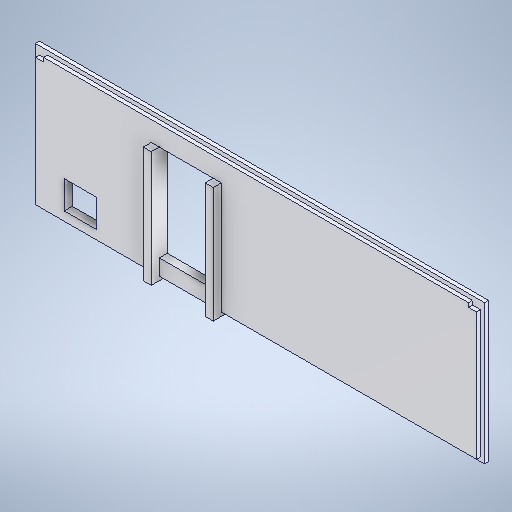
# Autodesk Inventor part: back
Saved by Autodesk Inventor 2025 (Build 290162000, 162)
## iProperties
Created: 2025-05-20
Part Number: back
Material: Generic
Document SubType Name: Modeling
Designer: ethan
Density: 1 g/cm^3
Appearance: PTFE
Author: ethan
Autodesk Inventor part; units mm, degrees
ref_plane "YZ Plane" through (0, 0, 0) normal (1, 0, 0) x (0, 1, 0)
ref_plane "XZ Plane" through (0, 0, 0) normal (0, 1, 0) x (-1, 0, 0)
ref_plane "XY Plane" through (0, 0, 0) normal (0, 0, 1) x (1, 0, 0)
sketch "Sketch1" plane through (0, 0, 0) normal (0, 0, 1) x (1, 0, 0)
  line L0 (0, 0) -> (224.6, 0)
  line L1 (224.6, 0) -> (224.6, 69.85)
  line L2 (224.6, 69.85) -> (0, 69.85)
  line L3 (0, 69.85) -> (0, 0)
  dimension "d0" = 224.6
  dimension "d1" = 69.85
  constraints: 8 end point, 2 parallel, 1 horizontal, 1 perpendicular
  measures "d0" distance of L2.end L1.end
  measures "d1" distance of L1.end L0.end
extrude "Extrusion1" add sketch "Sketch1" along normal blind 2
sketch "Sketch2" plane through (0, 0, 2) normal (0, 0, 1) x (1, 0, 0)
  line L0 (224.6, 0) -> (224.6, 69.85) projected
  line L1 (224.6, 69.85) -> (0, 69.85) projected
  line L2 (0, 69.85) -> (0, 0) projected
  line L3 (0, 0) -> (224.6, 0) projected
  line L4 (2, 67.85) -> (222.6, 67.85)
  line L5 (222.6, 67.85) -> (222.6, 2)
  line L6 (222.6, 2) -> (2, 2)
  line L7 (2, 2) -> (2, 67.85)
  dimension "d4" = 2
  constraints: 8 end point, 3 other
  measures "d4" distance between parallel lines of L1 L4
extrude "Extrusion2" add sketch "Sketch2" along normal blind 2 contours L4 L5 L6 L7
sketch "Sketch3" plane through (0, 0, 4) normal (0, 0, 1) x (1, 0, 0)
  line L0 (2, 2) -> (222.6, 2) construction
  line L1 (222.6, 2) -> (222.6, 67.85) construction
  line L2 (222.6, 67.85) -> (2, 67.85) construction
  line L3 (2, 67.85) -> (2, 2) construction
  line L4 (2, 67.85) -> (6, 67.85)
  line L5 (6, 67.85) -> (6, 65.85)
  line L6 (6, 65.85) -> (2, 65.85)
  line L7 (2, 65.85) -> (2, 67.85)
  line L8 (222.6, 67.85) -> (218.6, 67.85)
  line L9 (218.6, 67.85) -> (218.6, 65.85)
  line L10 (218.6, 65.85) -> (222.6, 65.85)
  line L11 (222.6, 65.85) -> (222.6, 67.85)
  point P0 (0, 0)
  dimension "d7" = 4
  dimension "d8" = 2
  dimension "d9" = 4
  dimension "d10" = 2
  constraints: 16 end point, 4 parallel, 2 horizontal, 2 perpendicular
  measures "d7" distance of L5.end L6.end
  measures "d8" distance of L4.end L5.end
  measures "d9" distance of L10.end L9.end
  measures "d10" distance of L9.end L8.end
extrude "Extrusion3" cut sketch "Sketch3" against normal blind 2
sketch "Sketch4" plane through (0, 0, 4) normal (0, 0, 1) x (1, 0, 0)
  line L0 (6, 67.85) -> (6, 65.85) construction
  line L1 (6, 65.85) -> (2, 65.85) construction
  line L2 (2, 65.85) -> (2, 2) construction
  line L3 (2, 2) -> (222.6, 2) construction
  line L4 (222.6, 2) -> (222.6, 65.85) construction
  line L5 (222.6, 65.85) -> (218.6, 65.85) construction
  line L6 (218.6, 65.85) -> (218.6, 67.85) construction
  line L7 (218.6, 67.85) -> (6, 67.85) construction
  line L8 (2, 2) -> (24.75, 2) construction
  line L9 (24.75, 2) -> (24.75, 13.5) construction
  line L10 (24.75, 13.5) -> (2, 13.5) construction
  line L11 (2, 13.5) -> (2, 2) construction
  line L12 (16.4203, 6.5) -> (32.4203, 6.5)
  line L13 (32.4203, 6.5) -> (32.4203, 20.5)
  line L14 (32.4203, 20.5) -> (16.4203, 20.5)
  line L15 (16.4203, 20.5) -> (16.4203, 6.5)
  line L16 (16.4203, 6.5) -> (32.4203, 20.5) construction
  line L17 (32.4203, 6.5) -> (16.4203, 20.5) construction
  point P0 (0, 0)
  point P1 (24.4203, 13.5)
  dimension "d13" = 22.75
  dimension "d14" = 11.5
  dimension "d15" = 16
  dimension "d16" = 14
  constraints: 20 end point, 4 parallel, 2 horizontal, 2 midpoint, 2 perpendicular, 1 point on line
  measures "d13" distance of L10.end L9.end
  measures "d14" distance of L9.end L8.end
  measures "d15" distance of L14.end L13.end
  measures "d16" distance of L13.end L12.end
extrude "Extrusion4" cut sketch "Sketch4" against normal up to surface (4 mm away)
sketch "Sketch5" plane through (0, 0, 4) normal (0, 0, 1) x (1, 0, 0)
  line L0 (32.4203, 20.5) -> (32.4203, 6.5) construction
  line L1 (32.4203, 6.5) -> (16.4203, 6.5) construction
  line L2 (16.4203, 6.5) -> (16.4203, 20.5) construction
  line L3 (16.4203, 20.5) -> (32.4203, 20.5) construction
  line L4 (6, 67.85) -> (6, 65.85) construction
  line L5 (6, 65.85) -> (2, 65.85) construction
  line L6 (2, 65.85) -> (2, 2) construction
  line L7 (2, 2) -> (222.6, 2) construction
  line L8 (222.6, 2) -> (222.6, 65.85) construction
  line L9 (222.6, 65.85) -> (218.6, 65.85) construction
  line L10 (218.6, 65.85) -> (218.6, 67.85) construction
  line L11 (218.6, 67.85) -> (6, 67.85) construction
  line L12 (32.4203, 20.5) -> (77.4203, 20.5) construction
  line L13 (63.9203, 9.925) -> (90.9203, 9.925)
  line L14 (90.9203, 9.925) -> (90.9203, 57.925)
  line L15 (90.9203, 57.925) -> (63.9203, 57.925)
  line L16 (63.9203, 57.925) -> (63.9203, 9.925)
  line L17 (63.9203, 9.925) -> (90.9203, 57.925) construction
  line L18 (90.9203, 9.925) -> (63.9203, 57.925) construction
  point P0 (0, 0)
  point P1 (77.4203, 33.925)
  dimension "d19" = 45
  dimension "d20" = 27
  dimension "d21" = 48
  constraints: 14 end point, 2 horizontal, 2 midpoint, 2 parallel, 1 perpendicular
  measures "d19" distance of L0.start L12.end
  measures "d20" distance of L15.end L14.end
  measures "d21" distance of L14.end L13.end
extrude "Extrusion5" cut sketch "Sketch5" against normal up to surface (4 mm away)
sketch "Sketch6" plane through (0, 0, 4) normal (0, 0, 1) x (1, 0, 0)
  line L0 (90.9203, 57.925) -> (90.9203, 9.925) construction
  line L1 (90.9203, 9.925) -> (63.9203, 9.925) construction
  line L2 (63.9203, 9.925) -> (63.9203, 57.925) construction
  line L3 (63.9203, 57.925) -> (90.9203, 57.925) construction
  line L4 (32.4203, 20.5) -> (32.4203, 6.5) construction
  line L5 (32.4203, 6.5) -> (16.4203, 6.5) construction
  line L6 (16.4203, 6.5) -> (16.4203, 20.5) construction
  line L7 (16.4203, 20.5) -> (32.4203, 20.5) construction
  line L8 (6, 67.85) -> (6, 65.85) construction
  line L9 (6, 65.85) -> (2, 65.85) construction
  line L10 (2, 65.85) -> (2, 2) construction
  line L11 (2, 2) -> (222.6, 2) construction
  line L12 (222.6, 2) -> (222.6, 65.85) construction
  line L13 (222.6, 65.85) -> (218.6, 65.85) construction
  line L14 (218.6, 65.85) -> (218.6, 67.85) construction
  line L15 (218.6, 67.85) -> (6, 67.85) construction
  line L16 (0, 0) -> (224.6, 0) construction
  line L17 (63.9203, 0) -> (59.9203, 0) construction
  line L18 (59.9203, 0) -> (59.9203, 57.925) construction
  line L19 (59.9203, 57.925) -> (63.9203, 57.925) construction
  line L20 (63.9203, 57.925) -> (63.9203, 0) construction
  line L21 (90.9203, 57.925) -> (94.9203, 57.925) construction
  line L22 (94.9203, 57.925) -> (94.9203, 0) construction
  line L23 (94.9203, 0) -> (90.9203, 0) construction
  line L24 (90.9203, 0) -> (90.9203, 57.925) construction
  line L25 (59.9203, 57.925) -> (63.9203, 57.925)
  line L26 (63.9203, 57.925) -> (63.9203, 0)
  line L27 (63.9203, 0) -> (59.9203, 0)
  line L28 (59.9203, 0) -> (59.9203, 57.925)
  line L29 (90.9203, 0) -> (94.9203, 0)
  line L30 (94.9203, 0) -> (94.9203, 57.925)
  line L31 (94.9203, 57.925) -> (90.9203, 57.925)
  line L32 (90.9203, 57.925) -> (90.9203, 0)
  dimension "d24" = 4
  dimension "d25" = 4
  constraints: 32 end point, 8 parallel, 4 horizontal, 4 perpendicular, 2 point on line
  measures "d24" distance of L18.end L19.end
  measures "d25" distance of L22.end L23.end
extrude "Extrusion6" add sketch "Sketch6" along normal blind 4 and the other way blind 2
body "Solid1"
